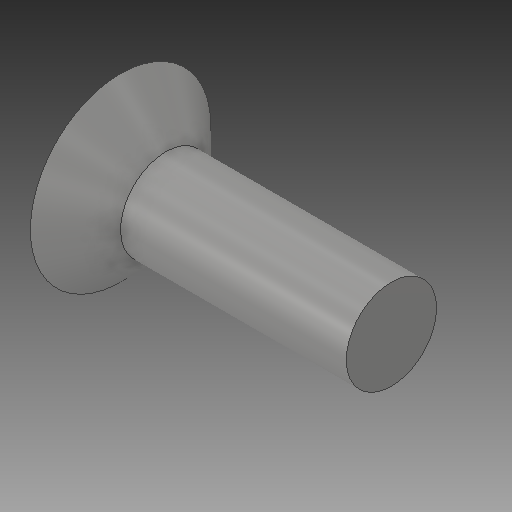
# Autodesk Inventor part: Parts_FlatScrew_M2_L6
Saved by Autodesk Inventor 2018.2 (Build 222227000, 227)
## iProperties
Part Number: Parts_FlatScrew_M2_L6
Material: 鋼
Document SubType Name: Modeling
Designer: sktom
Density: 7.85 g/cm^3
Appearance: プレート
Catalog Web Link: http://wilco.jp/products/F/FBF-N.html
Vendor: wilco
Author: sktom
Title: Parts_FlatScrew_M2_L6
Autodesk Inventor part; units mm, degrees
ref_plane "YZ Plane" through (0, 0, 0) normal (1, 0, 0) x (0, 1, 0)
ref_plane "XZ Plane" through (0, 0, 0) normal (0, 1, 0) x (-1, 0, 0)
ref_plane "XY Plane" through (0, 0, 0) normal (0, 0, 1) x (1, 0, 0)
sketch "スケッチ1" plane through (0, 0, 0) normal (0, 0, 1) x (1, 0, 0)
  line L0 (0, 0) -> (0, 2)
  line L1 (1, 1) -> (6, 1)
  line L2 (6, 1) -> (6, 0)
  line L3 (6, 0) -> (0, 0)
  line L4 (1, 1) -> (0, 2)
  dimension "d3" = 1
  dimension "d5" = 2
  dimension "d6" = 6
  dimension "d7" = 1
  constraints: 10 end point, 2 perpendicular, 1 vertical
  measures "d3" distance between parallel lines of L3 L1
  measures "d5" distance of L0.start L0.end
  measures "d6" distance between parallel lines of L0 L2
  measures "d7" distance from line of L0 L1.start
revolve "回転1" add sketch "スケッチ1" angle 360 about axis through (6, 0, 0) along (-1, 0, 0)
